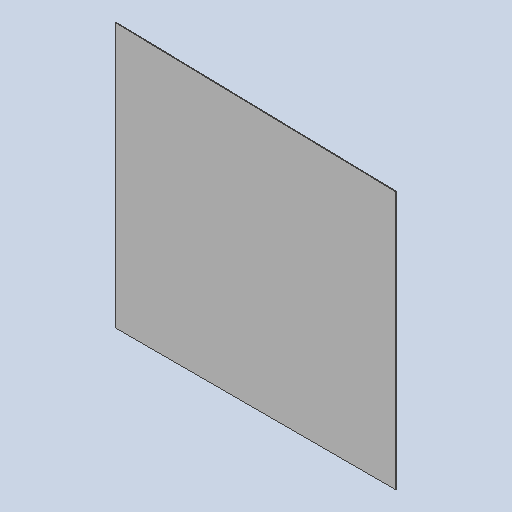
# Autodesk Inventor part: GBK 2133 shield 3
Saved by Autodesk Inventor 2026.2 (Build 302298000, 298)
## iProperties
Created: 2026-04-17
Part Number: GBK 2133 shield 3
Material: Steel
Document SubType Name: Sheet Metal
Designer: admin
Stock Number: 2133
Mass: 64094.5 g
Surface Area: 41053.3 cm^2
Volume: 8164.91 cm^3
Density: 7.85 g/cm^3
Sheet Metal Rule: Default_mm
Sheet Metal Width: 1396,000 mm
Sheet Metal Length: 1480,000 mm
Sheet Metal Area: 2066080,000 mm^2
Appearance: Default
Flat Pattern Width: 139.6 cm
Flat Pattern Length: 148 cm
Flat Pattern Area: 20660.8 cm^2
Project: 2
Author: admin
Autodesk Inventor part; units mm, degrees
ref_plane "YZ Plane" through (0, 0, 0) normal (1, 0, 0) x (0, 1, 0)
ref_plane "XZ Plane" through (0, 0, 0) normal (0, 1, 0) x (-1, 0, 0)
ref_plane "XY Plane" through (0, 0, 0) normal (0, 0, 1) x (1, 0, 0)
sketch "Sketch1" plane through (0, 0, 0) normal (0, 0, 1) x (1, 0, 0)
  line L0 (740, -745) -> (-740, -745)
  line L1 (-740, -745) -> (-740, 745)
  line L2 (-740, 745) -> (740, 745)
  line L3 (740, 745) -> (740, -745)
  line L4 (740, -745) -> (-740, 745) construction
  line L5 (-740, -745) -> (740, 745) construction
  line L6 (-740, 651) -> (740, 617.4141)
  point P0 (0, 0)
  dimension "d0" = 1480
  dimension "d1" = 1490
  dimension "d3" = 1.3
  dimension "d6" = 1396
  measures "d0" distance of L1.end L2.end
  measures "d1" distance of L0.end L1.end
  measures "d3" angle of L2 L6
  measures "d6" distance of L0.end L6.start
extrude "Plate1" add sketch "Sketch1" along normal blind 4 contours L0 L1 L6 L3
sketch "Sketch2" plane through (0, 0, 0) normal (0, 0, -1) x (-1, 0, 0)
  line L0 (499.781, -578.4604) -> (499.781, -902.2727) construction
  line L1 (499.781, -902.2727) -> (469.8587, -902.2727) construction
  line L2 (469.8587, -902.2727) -> (469.8587, -578.4604) construction
  line L3 (469.8587, -578.4604) -> (499.781, -578.4604) construction
  point P0 (0, 0)
  constraints: 2 other
mark "Mark1"
sketch "Эскиз3" plane through (0, 0, 0) normal (0, 0, -1) x (-1, 0, 0)
  line L0 (710, -489.5) -> (770, -489.5) projected
  line L1 (710, -489.5) -> (710, -485.5) projected
  line L2 (710, 7.1667) -> (770, 7.1667) projected
  line L3 (710, 7.1667) -> (710, 11.1667) projected
  line L4 (710, 503.8333) -> (770, 503.8333) projected
  line L5 (710, 503.8333) -> (710, 507.8333) projected
  line L6 (669.8628, -493) -> (669.8628, -590) projected
  line L7 (669.8628, -590) -> (665.8638, -590) projected
  line L8 (169.7342, -493) -> (169.7342, -590) projected
  line L9 (169.7342, -590) -> (165.7352, -590) projected
  line L10 (-330.3944, -493) -> (-330.3944, -590) projected
  line L11 (-330.3944, -590) -> (-334.3934, -590) projected
  line L12 (-738.6395, -489.5) -> (-680, -489.5) projected
  line L13 (-680, -489.5) -> (-680, -485.5) projected
  line L14 (-738.6395, 7.1667) -> (-680, 7.1667) projected
  line L15 (-680, 7.1667) -> (-680, 11.1667) projected
  line L16 (-738.6395, 503.8333) -> (-680, 503.8333) projected
  line L17 (-680, 503.8333) -> (-680, 507.8333) projected
  line L18 (169.7342, 715) -> (169.7342, 511.3333) projected
  line L19 (-330.3944, 715) -> (-330.3944, 511.3333) projected
  point P0 (0, 0)
mark "Маркировка2"
equation "\"d0\" = Лист_ширина"
equation "\"d2\" = Thickness"
equation "\"BendRadius\" = Thickness"
equation "\"BendReliefWidth\" = Thickness"
equation "\"BendReliefDepth\" = 0.5 * Thickness"
equation "\"CornerReliefSize\" = 4 * Thickness"
equation "\"MinimumRemnant\" = 2 * Thickness"
equation "\"TransitionRadius\" = BendRadius"
equation "\"JacobiRadiusSize\" = BendRadius"
equation "\"GapSize\" = Thickness"
equation "\"Лист_ширина\" = 1480"
equation "\"Thickness\" = 4"
body "Solid1"
